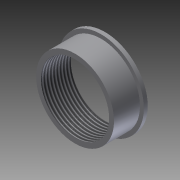
# Autodesk Inventor part: base_a
Saved by Autodesk Inventor 2011 (Build 150239000, 239)
## iProperties
Created: 2011-01-25
Part Number: base_a
Document SubType Name: Modeling
Designer: labuser
Density: 1 g/cm^3
Author: labuser
Autodesk Inventor part; units mm, degrees
ref_plane "YZ Plane" through (0, 0, 0) normal (1, 0, 0) x (0, 1, 0)
ref_plane "XZ Plane" through (0, 0, 0) normal (0, 1, 0) x (-1, 0, 0)
ref_plane "XY Plane" through (0, 0, 0) normal (0, 0, 1) x (1, 0, 0)
sketch "Sketch1" plane through (0, 0, 0) normal (0, 0, 1) x (1, 0, 0)
  circle A0 centre (0, 0) radius 8.382
  dimension "d0" = 16.764
  constraints: 1 centre point, 1 coincident
  measures "d0" diameter of A0
extrude "Extrusion1" add sketch "Sketch1" along normal blind 0.762
sketch "Sketch3" plane through (0, 0, 0.762) normal (0, 0, 1) x (1, 0, 0)
  circle A0 centre (0, 0) radius 8.382 projected
  circle A1 centre (0, 0) radius 7.62
  dimension "d13" = 15.24
  constraints: 1 centre point, 1 coincident
  measures "d13" diameter of A1
extrude "Extrusion2" add sketch "Sketch3" along normal blind 5.08 contours A1
sketch "Sketch4" plane through (0, 0, 5.842) normal (0, 0, 1) x (1, 0, 0)
  circle A0 centre (0, 0) radius 7.62 projected
  circle A1 centre (0, 0) radius 6.6675
  dimension "d16" = 13.335
  constraints: 1 centre point, 1 coincident
  measures "d16" diameter of A1
extrude "Extrusion3" cut sketch "Sketch4" against normal through all contours A1
thread "Thread2" size "4-40 UNC" class "2B" standard "ANSI Unified Screw Threads" full length
body "Solid1"
